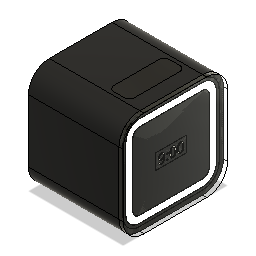
Sunrise_Alarm_V3_Idea (Autodesk Fusion 360 design; units mm, degrees)
Autodesk Fusion 360 part; units mm, degrees
sketch "Sketch1" plane through (0, 0, 0) normal (1, 0, 0) x (0, 0, -1)
  line L0 (0, 0) -> (-22.5, 0)
  line L1 (-37.5, 15) -> (-37.5, 60)
  line L2 (-22.5, 75) -> (0, 75)
  line L3 (0, 75) -> (0, 0)
  arc A0 (-22.5, 75) -> (-37.5, 60) centre (-22.5, 60) ccw
  arc A1 (-37.5, 15) -> (-22.5, 0) centre (-22.5, 15) ccw
  line L4 (0, 3) -> (-22.5, 3)
  arc A2 (-34.5, 15) -> (-22.5, 3) centre (-22.5, 15) ccw
  line L5 (-34.5, 15) -> (-34.5, 60)
  arc A3 (-22.5, 72) -> (-34.5, 60) centre (-22.5, 60) ccw
  line L6 (-22.5, 72) -> (0, 72)
  line L7 (37.5, 15) -> (37.5, 60)
  arc A4 (22.5, 3) -> (34.5, 15) centre (22.5, 15) ccw
  arc A5 (22.5, 0) -> (37.5, 15) centre (22.5, 15) ccw
  arc A6 (34.5, 60) -> (22.5, 72) centre (22.5, 60) ccw
  arc A7 (37.5, 60) -> (22.5, 75) centre (22.5, 60) ccw
  line L8 (34.5, 15) -> (34.5, 60)
  line L9 (22.5, 75) -> (0, 75)
  line L10 (22.5, 72) -> (0, 72)
  line L11 (0, 3) -> (22.5, 3)
  line L12 (0, 0) -> (22.5, 0)
  line L13 (22.5, 70) -> (0, 70)
  line L14 (-22.5, 70) -> (0, 70)
  arc A8 (-22.5, 70) -> (-32.5, 60) centre (-22.5, 60) ccw
  line L15 (-32.5, 15) -> (-32.5, 60)
  arc A9 (-32.5, 15) -> (-22.5, 5) centre (-22.5, 15) ccw
  line L16 (0, 5) -> (-22.5, 5)
  line L17 (0, 5) -> (22.5, 5)
  arc A10 (22.5, 5) -> (32.5, 15) centre (22.5, 15) ccw
  line L18 (32.5, 15) -> (32.5, 60)
  arc A11 (32.5, 60) -> (22.5, 70) centre (22.5, 60) ccw
  line L19 (-22.5, 65) -> (0, 65)
  line L20 (22.5, 65) -> (0, 65)
  arc A12 (27.5, 60) -> (22.5, 65) centre (22.5, 60) ccw
  line L21 (27.5, 15) -> (27.5, 60)
  arc A13 (22.5, 10) -> (27.5, 15) centre (22.5, 15) ccw
  line L22 (0, 10) -> (22.5, 10)
  line L23 (0, 10) -> (-22.5, 10)
  arc A14 (-27.5, 15) -> (-22.5, 10) centre (-22.5, 15) ccw
  line L24 (-27.5, 15) -> (-27.5, 60)
  arc A15 (-22.5, 65) -> (-27.5, 60) centre (-22.5, 60) ccw
  line L25 (11, 32) -> (-11, 32)
  line L26 (-11, 32) -> (-11, 43)
  line L27 (-11, 43) -> (11, 43)
  line L28 (11, 43) -> (11, 32)
  line L29 (11, 32) -> (-11, 43) construction
  line L30 (-11, 32) -> (11, 43) construction
  line L31 (-11, 32) -> (11, 32) construction
  line L32 (11, 32) -> (11, 43) construction
  line L33 (11, 43) -> (-11, 43) construction
  line L34 (-11, 43) -> (-11, 32) construction
  point P0 (-37.5, 0)
  point P1 (37.5, 0)
  point P2 (0, 37.5)
  dimension "d1" = 37.5
  dimension "d2" = 75
  dimension "d3" = 15
  dimension "d4" = 3
  dimension "d5" = -5
  dimension "d6" = 10
  dimension "d7" = 22
  dimension "d8" = 11
  dimension "d9" = 7
  text T0 "9:00" font "Arial" height 7 align centre middle in box 22 x 11 at (-11, 32) x (1, 0) y (0, 1) spacing 1
  constraint horizontal L0
  constraint vertical L1
  constraint horizontal L2
  constraint vertical L3
  constraint coincident L0.start L3.end
  constraint tangent L1 A0
  constraint tangent L2 A0
  constraint coincident P0 L0
  constraint coincident P0 L1
  constraint tangent L0 A1
  constraint tangent L1 A1
  constraint equal A0 A1
  constraint symmetric L0.start L3 L12.start
  constraint symmetric P0 L3 P1
  constraint symmetric L2.end L3 L9.end
  constraint symmetric L3 L1.end L7.end
  constraint symmetric L3 L2.start A7.end
  constraint symmetric L3 A0 A7
  constraint symmetric L3 L0.end A5.start
  constraint symmetric L3 L1.start L7.start
  constraint symmetric L3 A1 A5
  constraint symmetric L3 L4.start L11.start
  constraint symmetric L3 L4.end A4.start
  constraint symmetric L3 A2.start A4.end
  constraint symmetric L3 A2 A4
  constraint symmetric L3 L5.end A6.start
  constraint symmetric L3 A3.start A6.end
  constraint symmetric L3 A3 A6
  constraint symmetric L3 L6.end L10.end
  constraint horizontal L25
  constraint perpendicular L25 L26
  constraint parallel L25 L27
  constraint parallel L26 L28
  constraint coincident L29 P2
  constraint coincident L30 P2
  constraint midpoint L3 P2
  constraint coincident L25.start
  constraint coincident L26.end
  measures "d1" distance of L0.start P0
  measures "d2" distance of L0.start L2.end
  measures "d3" radius of A0
  measures "d7" distance of L26.end L27.end
  measures "d8" distance of L25.end L26.end
extrude "Extrude1" add sketch "Sketch1" sketch "Sketch1" along normal blind 3 of sketch 2 text T0 makes body 1
extrude "Extrude2" add sketch "Sketch1" against normal blind 0.2 separate body contours L3 L4 A2 L5 A3 L6 L14 A8 L15 A9 L16 | L3 A4 A6 L8 L10 L11 L13 L17 A10 L18 A11 makes body 2
extrude "Extrude3" add sketch "Sketch1" against normal blind 0.2 separate body contours L3 L19 L23 A14 L24 A15 L25 L26 L27 | L3 L20 A12 L21 A13 L22 L25 L27 L28 makes body 3
extrude "Extrude4" add sketch "Sketch1" against normal blind 0.2 separate body contours L3 L14 A8 L15 A9 L16 L19 L23 A14 L24 A15 | L3 L13 L17 A10 L18 A11 L20 A12 L21 A13 L22 makes body 4
extrude "Extrude5" add sketch "Sketch1" against normal blind 2 separate body contours L3 L25 L26 L27 | L3 L25 L27 L28 makes body 5
extrude "Extrude6" cut sketch "Sketch1" against normal blind 0.1 text T0 bodies 5
extrude "Extrude7" add sketch "Sketch1" against normal blind 65 separate body contours L0 L1 L2 L3 A0 A1 L4 A2 L5 A3 L6 | L3 L7 A4 A5 A6 A7 L8 L9 L10 L11 L12 makes body 6
sketch "Sketch2" plane through (0, 75, 0) normal (0, 1, 0) x (-1, 0, 0)
  line L0 (0, 22.5) -> (0, -22.5)
  line L1 (0, -22.5) -> (65, -22.5)
  line L2 (65, -22.5) -> (65, 22.5)
  line L3 (65, 22.5) -> (0, 22.5)
  line L4 (0, 0) -> (10, 0)
  line L5 (10, 0) -> (25, 0)
  line L6 (25, 0) -> (25, 16)
  line L7 (21, 20) -> (14, 20)
  line L8 (10, 16) -> (10, 0)
  arc A0 (25, 16) -> (21, 20) centre (21, 16) ccw
  arc A1 (14, 20) -> (10, 16) centre (14, 16) ccw
  line L9 (25, 0) -> (25, -16)
  arc A2 (21, -20) -> (25, -16) centre (21, -16) ccw
  line L10 (21, -20) -> (14, -20)
  arc A3 (10, -16) -> (14, -20) centre (14, -16) ccw
  line L11 (10, -16) -> (10, 0)
  point P0 (10, 20)
  dimension "d24" = 10
  dimension "d25" = 15
  dimension "d26" = 20
  dimension "d27" = 4
  constraint coincident L4.start origin
  constraint parallel L3 L4
  constraint horizontal L5
  constraint vertical L6
  constraint horizontal L7
  constraint vertical L8
  constraint tangent L6 A0
  constraint tangent L7 A0
  constraint coincident P0 L7
  constraint coincident P0 L8
  constraint tangent L7 A1
  constraint tangent L8 A1
  constraint equal A0 A1
  constraint symmetric L4.end L5 L8.end
  constraint symmetric L6.start L5 L9.start
  constraint symmetric L5 L6.end L9.end
  constraint symmetric L5 L7.start A2.start
  constraint symmetric L5 A0 A2
  constraint symmetric L5 L7.end L10.end
  constraint symmetric L5 L8.start A3.start
  constraint symmetric L5 A1 A3
  measures "d24" distance of L4.start L4.end
  measures "d25" distance of L4.end L5.end
  measures "d26" distance of L4.end P0
  measures "d27" radius of A0
extrude "Extrude8" cut sketch "Sketch2" against normal blind 1.7 contours L5 L6 L7 L8 A0 A1 | L5 L9 A2 L10 A3 L11 bodies 6
extrude "Extrude9" add sketch "Sketch2" against normal blind 1.7 separate body contours L5 L6 L7 L8 A0 A1 | L5 L9 A2 L10 A3 L11 makes body 7
equation "d1 = ( 75 / 2 ) * 1 mm"
named bodies: "Acrylic Front", "Black Vinyl 1", "Black Vinyl 2", "Frosted Vinyl", "Display", "Case"
